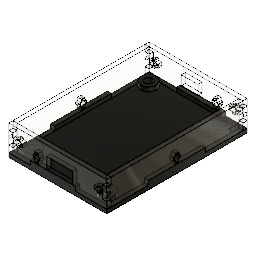
FinalProject_Enclosure_v2 (Autodesk Fusion 360 design; units mm, degrees)
Autodesk Fusion 360 part; units mm, degrees
(part 1 of 2)
sketch "Sketch1" plane through (0, 0, 0) normal (0, 0, 1) x (1, 0, 0) in component "Internals"
  line L0 (31.75, 47) -> (-31.75, 47)
  line L1 (-31.75, 47) -> (-31.75, -47)
  line L2 (-31.75, -47) -> (31.75, -47)
  line L3 (31.75, -47) -> (31.75, 47)
  line L4 (31.75, 47) -> (-31.75, -47) construction
  line L5 (-31.75, 47) -> (31.75, -47) construction
  line L6 (50.5, 1.5) -> (-50.5, 1.5) construction
  line L7 (-50.5, 1.5) -> (-50.5, -4.5) construction
  line L8 (-50.5, -4.5) -> (50.5, -4.5) construction
  line L9 (50.5, -4.5) -> (50.5, 1.5) construction
  line L10 (0, -50.5) -> (0, 50.5) construction
  point P0 (-33.75, 0)
  point P1 (33.75, 0)
  constraint horizontal L0
  constraint perpendicular L0 L1
  constraint parallel L0 L2
  constraint parallel L1 L3
  constraint coincident L4 origin
  constraint coincident L5 origin
  measures "d16" distance of L1.end L2.end
  measures "d17" distance of L0.end L1.end
extrude "Extrude1" add sketch "Sketch1" along normal blind 1.5 makes body 1 in component "Internals"
sketch "Sketch2" plane through (0, 0, 1.5) normal (0, 0, 1) x (-1, 0, 0) in component "Internals"
  line L0 (-31.75, 47) -> (-31.75, -47)
  line L1 (-31.75, -47) -> (31.75, -47)
  line L2 (31.75, -47) -> (31.75, 47)
  line L3 (31.75, 47) -> (-31.75, 47)
  line L4 (31.75, -41) -> (-31.75, -41) construction
  line L5 (25.75, -47) -> (25.75, 47) construction
  line L6 (0, -47) -> (0, 47) construction
  line L7 (31.75, 0) -> (-31.75, 0) construction
  line L8 (31.75, 41) -> (-31.75, 41) construction
  line L9 (-25.75, -47) -> (-25.75, 47) construction
  circle A0 centre (25.75, 41) radius 1.5
  circle A1 centre (-25.75, 41) radius 1.5
  circle A2 centre (-25.75, -41) radius 1.5
  circle A3 centre (25.75, -41) radius 1.5
  dimension "d20" = 6
  dimension "d21" = 6
  dimension "d22" = 3
  dimension "d23" = 3
  dimension "d24" = 3
  dimension "d25" = 3
  constraint coincident L2 L4.start
  constraint coincident L0 L4.end
  constraint perpendicular L0 L4
  constraint coincident L1 L5.start
  constraint coincident L3 L5.end
  constraint perpendicular L3 L5
  constraint midpoint L1 L6.start
  constraint midpoint L3 L6.end
  constraint midpoint L2 L7.start
  constraint midpoint L0 L7.end
  constraint symmetric L4.start L7 L8.start
  constraint symmetric L4.end L7 L8.end
  constraint symmetric L5.start L6 L9.start
  constraint symmetric L5.end L6 L9.end
  constraint coincident L5 A0.centre
  constraint coincident L8 A0.centre
  constraint coincident L9 A1.centre
  constraint coincident L8 A1.centre
  constraint coincident L9 A2.centre
  constraint coincident L4 A2.centre
  constraint coincident L5 A3.centre
  constraint coincident L4 A3.centre
  measures "d20" distance of L1 L4
  measures "d21" distance of L2 L5
  measures "d22" diameter of A0
  measures "d23" diameter of A1
  measures "d24" diameter of A2
  measures "d25" diameter of A3
extrude "Extrude2" add sketch "Sketch2" along normal blind 14 contours A0 | A1 | A2 | A3 bodies 1 in component "Internals"
sketch "Sketch3" plane through (0, 0, 15.5) normal (0, 0, 1) x (-1, 0, 0) in component "Internals"
  circle A0 centre (25.75, 41) radius 1.5
  line L0 (-31.75, -47) -> (31.75, -47)
  line L1 (31.75, -47) -> (31.75, 47)
  line L2 (31.75, 47) -> (-31.75, 47)
  line L3 (-31.75, 47) -> (-31.75, -47)
  line L4 (-31.75, -47) -> (31.75, 47) construction
  line L5 (31.75, -47) -> (-31.75, 47) construction
  dimension "d28" = 63.5
  dimension "d29" = 94
  constraint horizontal L0
  constraint perpendicular L0 L1
  constraint parallel L0 L2
  constraint parallel L1 L3
  constraint coincident L4 origin
  constraint coincident L5 origin
  measures "d28" distance of L1.end L2.end
  measures "d29" distance of L0.end L1.end
extrude "Extrude3" add sketch "Sketch3" along normal blind 1.5 contours A0 | L0 L1 L2 L3 bodies 1 in component "Internals"
sketch "Sketch4" plane through (0, 0, 17) normal (0, 0, 1) x (-1, 0, 0) in component "Internals"
  line L0 (-31.75, 47) -> (-31.75, -47)
  line L1 (-31.75, -47) -> (31.75, -47)
  line L2 (31.75, -47) -> (31.75, 47)
  line L3 (31.75, 47) -> (-31.75, 47)
  line L4 (0, 47) -> (0, -47) construction
  line L5 (-31.75, 0) -> (31.75, 0) construction
  line L6 (-31.75, 1) -> (31.75, 1) construction
  line L7 (-5, 47) -> (-5, -47) construction
  line L8 (-5, 1) -> (-17.1, 1)
  line L9 (-17.1, 1) -> (-17.1, 13.1)
  line L10 (-17.1, 13.1) -> (-5, 13.1)
  line L11 (-5, 13.1) -> (-5, 1)
  line L12 (-17.1, 27.2) -> (-5, 27.2)
  line L13 (-17.1, 15.1) -> (-17.1, 27.2)
  line L14 (-5, 15.1) -> (-17.1, 15.1)
  line L15 (-5, 27.2) -> (-5, 15.1)
  line L16 (-17.1, -13.1) -> (-17.1, -1)
  line L17 (-17.1, -1) -> (-5, -1)
  line L18 (-5, -1) -> (-5, -13.1)
  line L19 (-5, -13.1) -> (-17.1, -13.1)
  line L20 (-17.1, -15.1) -> (-5, -15.1)
  line L21 (-17.1, -27.2) -> (-17.1, -15.1)
  line L22 (-5, -27.2) -> (-17.1, -27.2)
  line L23 (-5, -15.1) -> (-5, -27.2)
  line L24 (17.1, 27.2) -> (5, 27.2)
  line L25 (17.1, 15.1) -> (17.1, 27.2)
  line L26 (5, 15.1) -> (17.1, 15.1)
  line L27 (5, 27.2) -> (5, 15.1)
  line L28 (5, 13.1) -> (5, 1)
  line L29 (5, -1) -> (5, -13.1)
  line L30 (5, -15.1) -> (5, -27.2)
  line L31 (5, -27.2) -> (17.1, -27.2)
  line L32 (17.1, -27.2) -> (17.1, -15.1)
  line L33 (17.1, -15.1) -> (5, -15.1)
  line L34 (5, -13.1) -> (17.1, -13.1)
  line L35 (17.1, -13.1) -> (17.1, -1)
  line L36 (17.1, -1) -> (5, -1)
  line L37 (17.1, 1) -> (17.1, 13.1)
  line L38 (17.1, 13.1) -> (5, 13.1)
  line L39 (5, 1) -> (17.1, 1)
  line L40 (13, -29.2) -> (9.1, -29.2)
  line L41 (9.1, -29.2) -> (9.1, -41.1)
  line L42 (9.1, -41.1) -> (13, -41.1)
  line L43 (13, -41.1) -> (13, -29.2)
  line L44 (11.05, -15.1) -> (11.05, -53.5543) construction
  line L45 (11.05, -29.2) -> (11.05, -41.1) construction
  dimension "d32" = 1
  dimension "d33" = 5
  dimension "d34" = 12.1
  dimension "d35" = 12.1
  dimension "d36" = 12.1
  dimension "d37" = 12.1
  dimension "d38" = 12.1
  dimension "d39" = 12.1
  dimension "d40" = 12.1
  dimension "d41" = 12.1
  dimension "d42" = 3.9
  dimension "d43" = 11.9
  dimension "d44" = 2
  constraint midpoint L3 L4.start
  constraint midpoint L1 L4.end
  constraint midpoint L0 L5.start
  constraint midpoint L2 L5.end
  constraint coincident L0 L6.start
  constraint coincident L2 L6.end
  constraint perpendicular L2 L6
  constraint coincident L3 L7.start
  constraint coincident L1 L7.end
  constraint perpendicular L1 L7
  constraint horizontal L8
  constraint vertical L9
  constraint horizontal L10
  constraint vertical L11
  constraint coincident L6 L8.start
  constraint coincident L7 L8.start
  constraint horizontal L14
  constraint vertical L13
  constraint horizontal L12
  constraint vertical L15
  constraint horizontal L19
  constraint vertical L16
  constraint horizontal L17
  constraint vertical L18
  constraint horizontal L22
  constraint vertical L21
  constraint horizontal L20
  constraint vertical L23
  constraint symmetric L4 L8.start L28.end
  constraint symmetric L4 L8.end L37.start
  constraint symmetric L4 L9.end L37.end
  constraint symmetric L4 L10.end L28.start
  constraint symmetric L4 L12.start L24.start
  constraint symmetric L4 L12.end L24.end
  constraint symmetric L4 L14.start L26.start
  constraint symmetric L4 L13.start L25.start
  constraint symmetric L4 L16.end L35.end
  constraint symmetric L4 L17.end L29.start
  constraint symmetric L4 L18.end L29.end
  constraint symmetric L4 L16.start L34.end
  constraint symmetric L4 L21.start L31.end
  constraint symmetric L4 L20.end L30.start
  constraint symmetric L4 L22.start L30.end
  constraint symmetric L4 L20.start L32.end
  constraint horizontal L40
  constraint vertical L41
  constraint horizontal L42
  constraint vertical L43
  constraint midpoint L33 L44.start
  constraint perpendicular L1 L44
  constraint midpoint L40 L45.start
  constraint midpoint L42 L45.end
  constraint collinear L44 L45
  measures "d32" distance of L5 L6
  measures "d33" distance of L4 L7
  measures "d34" distance of L8.start L8.end
  measures "d35" distance of L8.start L10.end
  measures "d36" distance of L14.start L13.start
  measures "d37" distance of L12.end L14.start
  measures "d38" distance of L18.end L16.start
  measures "d39" distance of L17.end L18.end
  measures "d40" distance of L21.start L22.start
  measures "d41" distance of L20.end L22.start
  measures "d42" distance of L40.start L40.end
  measures "d43" distance of L40.start L42.end
  measures "d44" distance of L31 L40
extrude "Extrude4" add sketch "Sketch4" along normal blind 5.2 contours L40 L41 L42 L43 bodies 1 in component "Internals"
extrude "Extrude5" add sketch "Sketch4" along normal blind 6.4 contours L8 L9 L10 L11 | L12 L13 L14 L15 | L16 L17 L18 L19 | L20 L21 L22 L23 | L24 L25 L26 L27 | L28 L37 L38 L39 | L29 L34 L35 L36 | L30 L31 L32 L33 bodies 1 in component "Internals"
sketch "Sketch1 (2)" plane through (-31.75, 0, 0) normal (-1, 0, 0) x (0, -1, 0) in component "Long Side"
  line L0 (-47, 15.5) -> (47, 15.5)
  line L1 (47, 15.5) -> (47, 17)
  line L2 (47, 17) -> (-47, 17)
  line L3 (-47, 17) -> (-47, 15.5)
  line L4 (50.5, 1.5) -> (-50.5, 1.5) construction
  line L5 (-50.5, 1.5) -> (-50.5, -4.5) construction
  line L6 (-50.5, -4.5) -> (50.5, -4.5) construction
  line L7 (50.5, -4.5) -> (50.5, 1.5) construction
  line L8 (50.5, 1.5) -> (50.5, 32.1442) construction
  line L9 (-50.5, 1.5) -> (-50.5, 33.8603) construction
  line L10 (-50.5, 1.5) -> (50.5, 1.5)
  line L11 (50.5, 1.5) -> (50.5, 17)
  line L12 (50.5, 17) -> (-50.5, 17)
  line L13 (-50.5, 17) -> (-50.5, 1.5)
  line L14 (-50.5, 1.5) -> (-20.41, 1.5)
  line L15 (-20.41, 1.5) -> (-20.41, -1.5)
  line L16 (-20.41, -1.5) -> (-50.5, -1.5)
  line L17 (-50.5, -1.5) -> (-50.5, 1.5)
  line L18 (0, 30) -> (0, -21) construction
  line L19 (50.5, 1.5) -> (20.41, 1.5)
  line L20 (20.41, 1.5) -> (20.41, -1.5)
  line L21 (20.41, -1.5) -> (50.5, -1.5)
  line L22 (50.5, -1.5) -> (50.5, 1.5)
  line L23 (-1.25, 1.5) -> (1.25, 1.5)
  line L24 (1.25, 1.5) -> (1.25, 8.5)
  line L25 (1.25, 8.5) -> (-1.25, 8.5)
  line L26 (-1.25, 8.5) -> (-1.25, 1.5)
  line L27 (-2.45, 6.3) -> (2.45, 6.3)
  line L28 (2.45, 6.3) -> (2.45, 4.4)
  line L29 (2.45, 4.4) -> (-2.45, 4.4)
  line L30 (-2.45, 4.4) -> (-2.45, 6.3)
  line L31 (50.5, 17) -> (47.5, 17)
  line L32 (47.5, 17) -> (47.5, 12.375)
  line L33 (47.5, 12.375) -> (50.5, 12.375)
  line L34 (50.5, 12.375) -> (50.5, 17)
  line L35 (50.5, -1.5) -> (47.5, -1.5)
  line L36 (47.5, -1.5) -> (47.5, 3.125)
  line L37 (47.5, 3.125) -> (50.5, 3.125)
  line L38 (50.5, 3.125) -> (50.5, -1.5)
  circle A0 centre (49, 7.75) radius 1.25
  line L39 (50.5, 12.375) -> (47.5, 3.125) construction
  line L40 (-50.5, -1.5) -> (-47.5, -1.5)
  line L41 (-47.5, -1.5) -> (-47.5, 3.125)
  line L42 (-47.5, 3.125) -> (-50.5, 3.125)
  line L43 (-50.5, 3.125) -> (-50.5, -1.5)
  line L44 (-50.5, 17) -> (-47.5, 17)
  line L45 (-47.5, 17) -> (-47.5, 12.375)
  line L46 (-47.5, 12.375) -> (-50.5, 12.375)
  line L47 (-50.5, 12.375) -> (-50.5, 17)
  line L48 (-47.5, 12.375) -> (-50.5, 3.125) construction
  circle A1 centre (-49, 7.75) radius 1.25
  point P0 (0, 1.5)
  point P1 (0, 4.4)
  dimension "d61" = 101
  dimension "d62" = 15.5
  dimension "d63" = 30.09
  dimension "d64" = 3
  dimension "d71" = 2.5
  dimension "d72" = 7
  dimension "d73" = 4.9
  dimension "d74" = 1.9
  dimension "d75" = 2.9
  dimension "d77" = 3
  dimension "d78" = 4.625
  dimension "d79" = 3
  dimension "d80" = 4.625
  dimension "d81" = 2.5
  dimension "d82" = 3
  dimension "d83" = 4.625
  dimension "d84" = 3
  dimension "d85" = 4.625
  dimension "d86" = 2.5
  constraint coincident L4.start L7.end
  constraint perpendicular L4 L8
  constraint coincident L4.end L5.start
  constraint perpendicular L4 L9
  constraint horizontal L10
  constraint vertical L11
  constraint horizontal L12
  constraint vertical L13
  constraint horizontal L14
  constraint vertical L15
  constraint horizontal L16
  constraint vertical L17
  constraint vertical L18
  constraint symmetric L4.end L18 L4.start
  constraint symmetric L14.end L18 L19.end
  constraint symmetric L15.end L18 L20.end
  constraint symmetric L16.end L18 L21.end
  constraint horizontal L23
  constraint vertical L24
  constraint horizontal L25
  constraint vertical L26
  constraint coincident L10 L23.start
  constraint midpoint L23 P0
  constraint midpoint L10 P0
  constraint horizontal L27
  constraint vertical L28
  constraint horizontal L29
  constraint vertical L30
  constraint midpoint L29 P1
  constraint coincident L18 P1
  constraint horizontal L31
  constraint vertical L32
  constraint horizontal L33
  constraint vertical L34
  constraint horizontal L35
  constraint vertical L36
  constraint horizontal L37
  constraint vertical L38
  constraint midpoint A0.centre L39
  constraint horizontal L40
  constraint vertical L41
  constraint horizontal L42
  constraint vertical L43
  constraint horizontal L44
  constraint vertical L45
  constraint horizontal L46
  constraint vertical L47
  constraint midpoint L48 A1.centre
  measures "d61" distance of L4.end L4.start
  measures "d62" distance of L4.end L12.end
  measures "d63" distance of L4.end L14.end
  measures "d64" distance of L4.end L16.end
  measures "d71" distance of L23.start L23.end
  measures "d72" distance of L23.start L25.end
  measures "d73" distance of L27.start L27.end
  measures "d74" distance of L27.start L29.end
  measures "d75" distance of L10 L29
  measures "d77" distance of L11.end L31.end
  measures "d78" distance of L11.end L33.end
  measures "d79" distance of L21.end L35.end
  measures "d80" distance of L21.end L37.end
  measures "d81" diameter of A0
  measures "d82" distance of L16.end L40.end
  measures "d83" distance of L16.end L42.end
  measures "d84" distance of L12.end L44.end
  measures "d85" distance of L12.end L46.end
  measures "d86" diameter of A1
extrude "Extrude1'" add sketch "Sketch1 (2)" along normal blind 3 from surface at 0.5 separate body contours L0 L1 L2 L3 L12 | L0 L1 L3 L10 L11 L12 L13 L14 L19 L24 L25 L26 L27 L28 L29 L30 L32 L33 L36 L37 L41 L42 L45 L46 | L10 L14 L15 L16 L41 | L10 L19 L20 L21 L36 makes body 2 in component "Long Side"
sketch "Sketch1 (3)" plane through (0, 0, 0) normal (0, 0, -1) x (1, 0, 0) in component "Base"
  line L0 (31.75, -47) -> (31.75, 47)
  line L1 (31.75, 47) -> (-31.75, 47)
  line L2 (-31.75, 47) -> (-31.75, -47)
  line L3 (-31.75, -47) -> (31.75, -47)
  line L4 (-32.25, -47.5) -> (32.25, -47.5)
  line L5 (32.25, -47.5) -> (32.25, 47.5)
  line L6 (32.25, 47.5) -> (-32.25, 47.5)
  line L7 (-32.25, 47.5) -> (-32.25, -47.5)
  line L8 (-32.25, -47.5) -> (32.25, 47.5) construction
  line L9 (32.25, -47.5) -> (-32.25, 47.5) construction
  line L10 (-35.25, -50.5) -> (35.25, -50.5)
  line L11 (35.25, -50.5) -> (35.25, 50.5)
  line L12 (35.25, 50.5) -> (-35.25, 50.5)
  line L13 (-35.25, 50.5) -> (-35.25, -50.5)
  line L14 (-35.25, -50.5) -> (35.25, 50.5) construction
  line L15 (35.25, -50.5) -> (-35.25, 50.5) construction
  dimension "d49_1" = 64.5
  dimension "d50_1" = 95
  dimension "d53_1" = 70.5
  dimension "d54_1" = 101
  constraint horizontal L4
  constraint perpendicular L4 L5
  constraint parallel L4 L6
  constraint parallel L5 L7
  constraint coincident L8 origin
  constraint coincident L9 origin
  constraint horizontal L10
  constraint perpendicular L10 L11
  constraint parallel L10 L12
  constraint parallel L11 L13
  constraint coincident L14 origin
  constraint coincident L15 origin
  measures "d49_1" distance of L5.end L6.end
  measures "d50_1" distance of L4.end L5.end
  measures "d53_1" distance of L11.end L12.end
  measures "d54_1" distance of L10.end L11.end
extrude "Extrude1''" add sketch "Sketch1 (3)" along normal blind 6 from surface at -1.5 separate body contours L10 L11 L12 L13 makes body 3 in component "Base"
extrude "Extrude2'" add sketch "Sketch1 (3)" along normal blind 3 from surface at 1.5 contours L0 L1 L2 L3 | L4 L5 L6 L7 bodies 3 in component "Base"
sketch "Sketch2 (2)" plane through (0, 0, 1.5) normal (0, 0, 1) x (-1, 0, 0) in component "Base"
  line L0 (32.25, 47.5) -> (32.25, -47.5)
  line L1 (32.25, -47.5) -> (-32.25, -47.5)
  line L2 (-32.25, -47.5) -> (-32.25, 47.5)
  line L3 (-32.25, 47.5) -> (32.25, 47.5)
  line L4 (35.25, -50.5) -> (35.25, 50.5)
  line L5 (35.25, 50.5) -> (-35.25, 50.5)
  line L6 (-35.25, 50.5) -> (-35.25, -50.5)
  line L7 (-35.25, -50.5) -> (35.25, -50.5)
  line L8 (32.25, -47.75) -> (32.25, -50.25)
  line L9 (32.25, 50.25) -> (32.25, 47.75)
  line L10 (32.25, -47.5) -> (32.25, 47.5)
  line L11 (32.25, 47.5) -> (32.25, 50.5)
  line L12 (32.25, 50.5) -> (32.25, 47.5)
  line L13 (32.25, 47.5) -> (32.25, 20.41)
  line L14 (32.25, 20.41) -> (32.25, 1.25)
  line L15 (32.25, 1.25) -> (32.25, 2.45)
  line L16 (32.25, 2.45) -> (32.25, 1.25)
  line L17 (32.25, 1.25) -> (32.25, -1.25)
  line L18 (32.25, -1.25) -> (32.25, -2.45)
  line L19 (32.25, -2.45) -> (32.25, -1.25)
  line L20 (32.25, -1.25) -> (32.25, -20.41)
  line L21 (32.25, -20.41) -> (32.25, -47.5)
  line L22 (32.25, -47.5) -> (32.25, -50.5)
  line L23 (32.25, -50.5) -> (32.25, -47.5)
  line L24 (35.25, -50.5) -> (32.25, -50.5)
  line L25 (32.25, -50.5) -> (32.25, -20.41)
  line L26 (32.25, -20.41) -> (35.25, -20.41)
  line L27 (35.25, -20.41) -> (35.25, -50.5)
  line L28 (35.25, 50.5) -> (32.25, 50.5)
  line L29 (32.25, 50.5) -> (32.25, 20.41)
  line L30 (32.25, 20.41) -> (35.25, 20.41)
  line L31 (35.25, 20.41) -> (35.25, 50.5)
  line L32 (35.25, -20.41) -> (32.25, 20.41) construction
  circle A0 centre (33.75, 0) radius 1.25
  line L33 (0, -50.5) -> (0, 50.5) construction
  line L34 (32.25, -20.41) -> (-35.25, -20.41) construction
  line L35 (32.25, 20.41) -> (-35.25, 20.41) construction
  line L36 (-35.25, -50.5) -> (-32.25, -50.5)
  line L37 (-32.25, -50.5) -> (-32.25, -20.41)
  line L38 (-32.25, -20.41) -> (-35.25, -20.41)
  line L39 (-35.25, -20.41) -> (-35.25, -50.5)
  line L40 (-35.25, 50.5) -> (-32.25, 50.5)
  line L41 (-32.25, 50.5) -> (-32.25, 20.41)
  line L42 (-32.25, 20.41) -> (-35.25, 20.41)
  line L43 (-35.25, 20.41) -> (-35.25, 50.5)
  line L44 (-35.25, -20.41) -> (-32.25, 20.41) construction
  circle A1 centre (-33.75, 0) radius 1.25
  line L45 (-35.25, -50.5) -> (-19.75, -50.5)
  line L46 (-19.75, -50.5) -> (-19.75, -47.5)
  line L47 (-19.75, -47.5) -> (-35.25, -47.5)
  line L48 (-35.25, -47.5) -> (-35.25, -50.5)
  line L49 (35.25, -50.5) -> (12.75, -50.5)
  line L50 (12.75, -50.5) -> (12.75, -47.5)
  line L51 (12.75, -47.5) -> (35.25, -47.5)
  line L52 (35.25, -47.5) -> (35.25, -50.5)
  line L53 (-35.25, 50.5) -> (-12.75, 50.5)
  line L54 (-12.75, 50.5) -> (-12.75, 47.5)
  line L55 (-12.75, 47.5) -> (-35.25, 47.5)
  line L56 (-35.25, 47.5) -> (-35.25, 50.5)
  line L57 (35.25, 50.5) -> (19.75, 50.5)
  line L58 (19.75, 50.5) -> (19.75, 47.5)
  line L59 (19.75, 47.5) -> (35.25, 47.5)
  line L60 (35.25, 47.5) -> (35.25, 50.5)
  circle A2 centre (-15.25, -49) radius 1.25
  circle A3 centre (15.25, 49) radius 1.25
  point P0 (35.25, -20.41)
  dimension "d90" = 2.5
  dimension "d91" = 2.5
  dimension "d121" = 15.5
  dimension "d122" = 3
  dimension "d123" = 22.5
  dimension "d124" = 3
  dimension "d125" = 22.5
  dimension "d126" = 3
  dimension "d127" = 15.5
  dimension "d128" = 3
  dimension "d129" = 2.5
  dimension "d130" = 2.5
  dimension "d150" = 4.5
  dimension "d151" = 4.5
  constraint horizontal L24
  constraint vertical L25
  constraint horizontal L26
  constraint vertical L27
  constraint coincident L20.end L21.start
  constraint coincident L4.start L7.end
  constraint horizontal L28
  constraint vertical L29
  constraint horizontal L30
  constraint vertical L31
  constraint coincident L13.end L14.start
  constraint coincident L4.end L5.start
  constraint coincident P0 L26.end
  constraint midpoint L32 A0.centre
  constraint midpoint L7 L33.start
  constraint midpoint L5 L33.end
  constraint coincident L6 L34.end
  constraint perpendicular L6 L34
  constraint coincident L6 L35.end
  constraint perpendicular L6 L35
  constraint horizontal L36
  constraint vertical L37
  constraint horizontal L38
  constraint vertical L39
  constraint coincident L2 L37.end
  constraint coincident L34 L37.end
  constraint coincident L6.end L7.start
  constraint horizontal L40
  constraint vertical L41
  constraint horizontal L42
  constraint vertical L43
  constraint coincident L35 L41.end
  constraint coincident L2 L41.end
  constraint coincident L5.end L6.start
  constraint midpoint L44 A1.centre
  constraint horizontal L45
  constraint vertical L46
  constraint horizontal L47
  constraint vertical L48
  constraint horizontal L49
  constraint vertical L50
  constraint horizontal L51
  constraint vertical L52
  constraint horizontal L53
  constraint vertical L54
  constraint horizontal L55
  constraint vertical L56
  constraint horizontal L57
  constraint vertical L58
  constraint horizontal L59
  constraint vertical L60
  measures "d90" diameter of A0
  measures "d91" diameter of A1
  measures "d121" distance of L6.end L45.end
  measures "d122" distance of L6.end L47.end
  measures "d123" distance of L4.start L49.end
  measures "d124" distance of L4.start L51.end
  measures "d125" distance of L5.end L53.end
  measures "d126" distance of L5.end L55.end
  measures "d127" distance of L4.end L57.end
  measures "d128" distance of L4.end L59.end
  measures "d129" diameter of A2
  measures "d130" diameter of A3
  measures "d150" distance of L46 A2.centre
  measures "d151" distance of L58 A3.centre
extrude "Extrude3'" cut sketch "Sketch2 (2)" against normal blind 3 contours L0 L4 L10 L13 L29 L30 L31 L59 | L3 L5 L9 L11 L12 L29 L57 L58 L59 | L4 L5 L9 L11 L12 L28 L29 L31 L57 L59 L60 | L3 L5 L41 L53 L54 L55 | L0 L4 L10 L21 L25 L26 L27 L51 | L5 L6 L40 L41 L43 L53 L55 L56 | L2 L6 L41 L42 L43 L55 | L4 L7 L8 L22 L23 L24 L25 L27 L49 L51 L52 | L1 L7 L8 L22 L23 L25 L49 L50 L51 | L2 L6 L37 L38 L39 L47 | L1 L7 L37 L45 L46 L47 | L6 L7 L36 L37 L39 L45 L47 L48 bodies 3 in component "Base"
extrude "Extrude4'" cut sketch "Sketch2 (2)" against normal blind 14 contours A0 | A1 | A2 | A3 bodies 3 in component "Base"
sketch "Sketch1 (4)" plane through (0, 47, 0) normal (0, 1, 0) x (-1, 0, 0) in component "Short Side"
  line L0 (-31.75, 15.5) -> (31.75, 15.5)
  line L1 (31.75, 15.5) -> (31.75, 17)
  line L2 (31.75, 17) -> (-31.75, 17)
  line L3 (-31.75, 17) -> (-31.75, 15.5)
  line L4 (12.75, 1.5) -> (-19.75, 1.5)
  line L5 (-19.75, -1.5) -> (-35.25, -1.5)
  line L6 (-35.25, -1.5) -> (-35.25, -4.5)
  line L7 (-35.25, -4.5) -> (35.25, -4.5)
  line L8 (35.25, -4.5) -> (35.25, -1.5)
  line L9 (35.25, -1.5) -> (12.75, -1.5)
  line L10 (35.25, -4.5) -> (35.25, 23) construction
  line L11 (-35.25, -1.5) -> (35.25, -1.5)
  line L12 (35.25, -1.5) -> (35.25, 17)
  line L13 (35.25, 17) -> (-35.25, 17)
  line L14 (-35.25, 17) -> (-35.25, -1.5)
  line L15 (35.25, 17) -> (32.25, 17)
  line L16 (32.25, 12.195) -> (35.25, 12.195)
  line L17 (35.25, 12.195) -> (35.25, 17)
  line L18 (35.25, -1.5) -> (32.25, -1.5)
  line L19 (32.25, 3.305) -> (35.25, 3.305)
  line L20 (35.25, 3.305) -> (35.25, -1.5)
  line L21 (-35.25, 17) -> (-32.25, 17)
  line L22 (-32.25, 12.195) -> (-35.25, 12.195)
  line L23 (-35.25, 12.195) -> (-35.25, 17)
  line L24 (-35.25, -1.5) -> (-32.25, -1.5)
  line L25 (-32.2728, 3.305) -> (-35.25, 3.305)
  line L26 (-35.25, 3.305) -> (-35.25, -1.5)
  line L27 (-32.2728, 3.305) -> (-35.25, 3.305)
  line L28 (-35.25, 3.305) -> (-35.25, 12.195)
  line L29 (-35.25, 12.195) -> (-32.2728, 12.195)
  line L30 (-32.2728, 12.195) -> (-32.2728, 3.305)
  line L31 (32.25, 3.305) -> (35.25, 3.305)
  line L32 (35.25, 3.305) -> (35.25, 12.195)
  line L33 (35.25, 12.195) -> (32.25, 12.195)
  line L34 (32.25, 12.195) -> (32.25, 3.305)
  line L35 (0.4382, 30) -> (0.4382, -14) construction
  line L36 (-9.5349, -1.5) -> (15.25, -1.5)
  line L37 (-0.8118, -1) -> (1.6882, -1)
  line L38 (35.25, 7.75) -> (-35.25, 7.75) construction
  line L39 (-32.2728, 9) -> (-25.2728, 9)
  line L40 (-25.2728, 9) -> (-25.2728, 6.5)
  line L41 (-25.2728, 6.5) -> (-32.2728, 6.5)
  line L42 (-32.2728, 6.5) -> (-32.2728, 9)
  line L43 (-27.4728, 10.2) -> (-29.3728, 10.2)
  line L44 (-29.3728, 10.2) -> (-29.3728, 5.3)
  line L45 (-29.3728, 5.3) -> (-27.4728, 5.3)
  line L46 (-27.4728, 5.3) -> (-27.4728, 10.2)
  line L47 (-27.4728, 10.2) -> (-29.3728, 5.3) construction
  line L48 (-29.3728, 10.2) -> (-27.4728, 5.3) construction
  line L49 (33.1492, 9) -> (26.1492, 9)
  line L50 (26.1492, 6.5) -> (33.1492, 6.5)
  line L51 (26.1492, 9) -> (26.1492, 6.5)
  line L52 (28.3492, 5.3) -> (28.3492, 10.2)
  line L53 (30.2492, 10.2) -> (30.2492, 5.3)
  line L54 (28.3492, 10.2) -> (30.2492, 10.2)
  line L55 (30.2492, 5.3) -> (28.3492, 5.3)
  line L56 (12.75, -1.5) -> (12.75, 1.5)
  line L57 (-19.75, 1.5) -> (-19.75, -1.5)
  line L58 (-15.25, 17) -> (-15.25, -1.5) construction
  line L59 (-19.66, 17) -> (-19.66, -1.5) construction
  line L60 (12.66, 17) -> (12.66, -1.5) construction
  line L61 (-14, 8.5) -> (-16.5, 8.5)
  line L62 (-16.5, 8.5) -> (-16.5, 1.5)
  line L63 (-16.5, 1.5) -> (-14, 1.5)
  line L64 (-14, 1.5) -> (-14, 8.5)
  line L65 (-14, 8.5) -> (-16.5, 1.5) construction
  line L66 (-16.5, 8.5) -> (-14, 1.5) construction
  line L67 (-12.8, 6.3) -> (-17.7, 6.3)
  line L68 (-17.7, 6.3) -> (-17.7, 4.4)
  line L69 (-17.7, 4.4) -> (-12.8, 4.4)
  line L70 (-12.8, 4.4) -> (-12.8, 6.3)
  line L71 (-12.8, 6.3) -> (-17.7, 4.4) construction
  line L72 (-17.7, 6.3) -> (-12.8, 4.4) construction
  line L73 (-2.75, 11) -> (9.25, 11)
  line L74 (9.25, 11) -> (9.25, 4)
  line L75 (9.25, 4) -> (-2.75, 4)
  line L76 (-2.75, 4) -> (-2.75, 11)
  line L77 (12.66, 1.5) -> (-19.66, 1.5)
  line L78 (-19.66, 1.5) -> (-19.66, -1.5)
  line L79 (-19.66, -1.5) -> (12.66, -1.5)
  line L80 (12.66, -1.5) -> (12.66, 1.5)
  point P0 (0.4382, -1)
  point P1 (0.4382, 5.5)
  point P2 (-32.2728, 7.75)
  point P3 (-28.4228, 7.75)
  point P4 (-15.25, 5)
  point P5 (-15.25, 1.5)
  point P6 (-15.25, 5.35)
  dimension "d96" = 70.5
  dimension "d97" = 18.5
  dimension "d98" = 3
  dimension "d99" = 4.805
  dimension "d100" = 3
  dimension "d101" = 4.805
  dimension "d102" = 3
  dimension "d103" = 4.805
  dimension "d104" = 3
  dimension "d105" = 4.805
  dimension "d108" = 2.5
  dimension "d113" = 7
  dimension "d114" = 2.5
  dimension "d115" = 1.9
  dimension "d116" = 4.9
  dimension "d117" = 2.9
  dimension "d152" = 20
  dimension "d153" = 15.59
  dimension "d154" = 22.59
  dimension "d155" = 7
  dimension "d156" = 4.9
  dimension "d157" = 1.9
  dimension "d159" = 12
  dimension "d160" = 7
  dimension "d162" = 26
  dimension "d163" = 32.5
  dimension "d180" = 6
  dimension "d184" = 2.9
  dimension "d185" = 2.5
  constraint coincident L7.end L8.start
  constraint perpendicular L7 L10
  constraint horizontal L11
  constraint vertical L12
  constraint horizontal L13
  constraint vertical L14
  constraint coincident L5.end L6.start
  constraint horizontal L15
  constraint horizontal L16
  constraint vertical L17
  constraint horizontal L18
  constraint horizontal L19
  constraint vertical L20
  constraint coincident L8.end L9.start
  constraint horizontal L21
  constraint horizontal L22
  constraint vertical L23
  constraint horizontal L24
  constraint horizontal L25
  constraint vertical L26
  constraint horizontal L27
  constraint vertical L28
  constraint horizontal L29
  constraint vertical L30
  constraint horizontal L31
  constraint vertical L32
  constraint horizontal L33
  constraint vertical L34
  constraint vertical L35
  constraint horizontal L36
  constraint coincident L11 L36.start
  constraint horizontal L37
  constraint midpoint L37 P0
  constraint vertical L35.end P0
  constraint coincident L35 P1
  constraint midpoint L12 L38.start
  constraint midpoint L28 L38.end
  constraint horizontal L39
  constraint vertical L40
  constraint horizontal L41
  constraint vertical L42
  constraint coincident L30 L39.start
  constraint midpoint L42 P2
  constraint horizontal L38.end P2
  constraint horizontal L43
  constraint perpendicular L43 L44
  constraint parallel L43 L45
  constraint parallel L44 L46
  constraint coincident L47 P3
  constraint coincident L48 P3
  constraint coincident L38 P3
  constraint symmetric L35 L39.start L49.start
  constraint symmetric L35 L39.end L49.end
  constraint symmetric L35 L40.end L50.start
  constraint symmetric L35 L41.end L50.end
  constraint symmetric L35 L43.start L52.end
  constraint symmetric L35 L43.end L53.start
  constraint symmetric L35 L44.end L53.end
  constraint symmetric L35 L45.end L52.start
  constraint coincident L13 L58.start
  constraint coincident L11 L58.end
  constraint perpendicular L11 L58
  constraint coincident L2 L59.start
  constraint coincident L11 L59.end
  constraint perpendicular L11 L59
  constraint coincident L13 L60.start
  constraint coincident L36 L60.end
  constraint perpendicular L36 L60
  constraint horizontal L61
  constraint perpendicular L61 L62
  constraint parallel L61 L63
  constraint parallel L62 L64
  constraint coincident L65 P4
  constraint coincident L66 P4
  constraint coincident L58 P4
  constraint coincident L63 P5
  constraint horizontal L67
  constraint perpendicular L67 L68
  constraint parallel L67 L69
  constraint parallel L68 L70
  constraint coincident L71 P6
  constraint coincident L72 P6
  constraint coincident L58 P6
  constraint horizontal L73
  constraint vertical L74
  constraint horizontal L75
  constraint vertical L76
  constraint horizontal L77
  constraint vertical L78
  constraint horizontal L79
  constraint vertical L80
  constraint coincident L60 L77.start
  constraint coincident L4 L77.start
  measures "d96" distance of L5.end L8.end
  measures "d97" distance of L5.end L13.end
  measures "d98" distance of L12.end L15.end
  measures "d99" distance of L12.end L16.end
  measures "d100" distance of L8.end L18.end
  measures "d101" distance of L8.end L19.end
  measures "d102" distance of L13.end L21.end
  measures "d103" distance of L13.end L22.end
  measures "d104" distance of L5.end L24.end
  measures "d105" distance of L5.end L25.end
  measures "d108" distance of L37.start L37.end
  measures "d113" distance of L39.start L39.end
  measures "d114" distance of L39.start L41.end
  measures "d115" distance of L44.end L45.end
  measures "d116" distance of L43.end L44.end
  measures "d117" distance of L30 L44
  measures "d152" distance of L14 L58
  measures "d153" distance of L23 L59
  measures "d154" distance of L10 L60
  measures "d155" distance of L61.end L62.end
  measures "d156" distance of L68.end L69.end
  measures "d157" distance of L67.end L68.end
  measures "d159" distance of L73.start L73.end
  measures "d160" distance of L73.start L75.end
  measures "d162" distance of L12 L74
  measures "d163" distance of L23 L76
  measures "d180" distance of L13 L73
  measures "d184" distance of L69.end L77
  measures "d185" distance of L61.start L61.end
sketch "Sketch3 (2)" plane through (0, 0, -1.5) normal (0, 0, 1) x (-1, 0, 0) in component "Base"
  line L0 (19.75, 47.5) -> (-12.75, 47.5)
  line L1 (-12.75, 47.5) -> (-12.75, 50.5)
  line L2 (-12.75, 50.5) -> (-35.25, 50.5)
  line L3 (-35.25, 50.5) -> (-35.25, 20.41)
  line L4 (-35.25, 20.41) -> (-32.25, 20.41)
  line L5 (-32.25, 20.41) -> (-32.25, -20.41)
  line L6 (-32.25, -20.41) -> (-35.25, -20.41)
  line L7 (-35.25, -20.41) -> (-35.25, -50.5)
  line L8 (-35.25, -50.5) -> (-19.75, -50.5)
  line L9 (-19.75, -50.5) -> (-19.75, -47.5)
  line L10 (-19.75, -47.5) -> (12.75, -47.5)
  line L11 (12.75, -47.5) -> (12.75, -50.5)
  line L12 (12.75, -50.5) -> (35.25, -50.5)
  line L13 (35.25, -50.5) -> (35.25, -20.41)
  line L14 (35.25, -20.41) -> (32.25, -20.41)
  line L15 (32.25, -20.41) -> (32.25, 20.41)
  line L16 (32.25, 20.41) -> (35.25, 20.41)
  line L17 (35.25, 20.41) -> (35.25, 50.5)
  line L18 (35.25, 50.5) -> (19.75, 50.5)
  line L19 (19.75, 50.5) -> (19.75, 47.5)
  circle A0 centre (-26.75, 41.5) radius 5.5
  line L20 (-12.75, 47.5) -> (-35.25, 47.5)
  line L21 (-32.25, 50.5) -> (-32.25, 20.41)
  line L22 (15.25, 49) -> (-15.25, -49) construction
  line L23 (-33.75, 0) -> (33.75, 0) construction
  line L24 (0, -50.5) -> (0, 50.5) construction
  circle A1 centre (26.75, 41.5) radius 5.5
  circle A2 centre (26.75, -41.5) radius 5.5
  circle A3 centre (-26.75, -41.5) radius 5.5
  circle A4 centre (-26.75, 41.5) radius 2.75
  circle A5 centre (26.75, 41.5) radius 2.75
  circle A6 centre (26.75, -41.5) radius 2.75
  circle A7 centre (-26.75, -41.5) radius 2.75
  line L25 (19.75, 47.5) -> (35.25, 47.5)
  line L26 (32.25, 20.41) -> (32.25, 50.5)
  line L27 (32.25, -20.41) -> (32.25, -50.5)
  line L28 (12.75, -47.5) -> (35.25, -47.5)
  line L29 (-19.75, -47.5) -> (-35.25, -47.5)
  line L30 (-32.25, -20.41) -> (-32.25, -50.5)
  line L31 (-32.25, 41.5) -> (-32.25, 50.5)
  line L32 (-26.75, 41.5) -> (-26.75, 47) construction
  line L33 (-26.75, 47) -> (-35.25, 47)
  line L34 (26.75, 47) -> (35.25, 47)
  line L35 (32.25, 41.5) -> (32.25, 50.5)
  line L36 (-26.75, -47) -> (-35.25, -47)
  line L37 (-32.25, -41.5) -> (-32.25, -50.5)
  line L38 (26.75, -47) -> (35.25, -47)
  line L39 (32.25, -41.5) -> (32.25, -50.5)
  point P0 (15.25, 49)
  point P1 (-33.75, 0)
  point P2 (-15.25, -49)
  point P3 (33.75, 0)
  dimension "d133" = 11
  dimension "d134" = 6
  dimension "d135" = 5.5
  dimension "d136" = 5.5
  constraint coincident P0 L22.start
  constraint coincident P2 L22.end
  constraint coincident P1 L23.start
  constraint coincident P3 L23.end
  constraint symmetric A0 L24 A1
  constraint symmetric A0 L23 A3
  constraint symmetric L23 A1 A2
  constraint concentric A0 A4
  constraint symmetric L24 A4 A5
  constraint symmetric L23 A4 A7
  constraint symmetric L23 A5 A6
  constraint coincident L0.start L19.end
  constraint coincident L17 L25.end
  constraint perpendicular L17 L25
  constraint coincident L15.end L16.start
  constraint coincident L18 L26.end
  constraint perpendicular L18 L26
  constraint coincident L14.end L15.start
  constraint coincident L12 L27.end
  constraint perpendicular L12 L27
  constraint coincident L10.end L11.start
  constraint coincident L13 L28.end
  constraint perpendicular L13 L28
  constraint coincident L9.end L10.start
  constraint coincident L7 L29.end
  constraint perpendicular L7 L29
  constraint coincident L5.end L6.start
  constraint coincident L8 L30.end
  constraint perpendicular L8 L30
  constraint coincident A0 L31.start
  constraint coincident L21.start L31.end
  constraint tangent A0 L31
  constraint coincident A0.centre A4.centre
  constraint coincident A0 L32.end
  constraint vertical L32
  constraint coincident L3 L33.end
  constraint perpendicular L3 L33
  constraint symmetric L24 L31.start L35.start
  constraint symmetric L24 L21.start L26.end
  constraint symmetric L24 L32.end L34.start
  constraint symmetric L24 L33.end L34.end
  constraint symmetric L23 L31.start L37.start
  constraint symmetric L23 L21.start L30.end
  constraint symmetric L23 L32.end L36.start
  constraint symmetric L23 L33.end L36.end
  constraint symmetric L23 L34.start L38.start
  constraint symmetric L23 L34.end L38.end
  constraint symmetric L23 L35.start L39.start
  constraint symmetric L23 L26.end L27.end
  measures "d133" diameter of A0
  measures "d134" distance of A0.centre L20
  measures "d135" distance of A0.centre L21
  measures "d136" diameter of A4
sketch "Sketch1 (5)" plane through (0, 47, 0) normal (0, 1, 0) x (-1, 0, 0) in component "Short Side v1"
  line L0 (-31.75, 15.5) -> (31.75, 15.5)
  line L1 (31.75, 15.5) -> (31.75, 17)
  line L2 (31.75, 17) -> (-31.75, 17)
  line L3 (-31.75, 17) -> (-31.75, 15.5)
  line L4 (-35.25, -1.5454) -> (-35.25, -4.5)
  line L5 (-35.25, -4.5) -> (35.25, -4.5)
  line L6 (35.25, -4.5) -> (35.25, -1.5)
  line L7 (35.25, -4.5) -> (35.25, 23) construction
  line L8 (-35.25, -1.5454) -> (35.25, -1.5454)
  line L9 (35.25, -1.5454) -> (35.25, 16.9546)
  line L10 (35.25, 16.9546) -> (-35.25, 16.9546)
  line L11 (-35.25, 16.9546) -> (-35.25, -1.5454)
  line L12 (35.25, 16.9546) -> (32.25, 16.9546)
  line L13 (32.25, 12.1496) -> (35.25, 12.1496)
  line L14 (35.25, 12.1496) -> (35.25, 16.9546)
  line L15 (35.25, -1.5) -> (32.25, -1.5)
  line L16 (32.25, 3.305) -> (35.25, 3.305)
  line L17 (35.25, 3.305) -> (35.25, -1.5)
  line L18 (-35.25, 16.9546) -> (-32.25, 16.9546)
  line L19 (-32.25, 12.1496) -> (-35.25, 12.1496)
  line L20 (-35.25, 12.1496) -> (-35.25, 16.9546)
  line L21 (-35.25, -1.5454) -> (-32.25, -1.5454)
  line L22 (-32.3728, 3.2596) -> (-35.25, 3.2596)
  line L23 (-35.25, 3.2596) -> (-35.25, -1.5454)
  line L24 (-32.3728, 3.2596) -> (-35.25, 3.2596)
  line L25 (-35.25, 3.2596) -> (-35.25, 12.1496)
  line L26 (-35.25, 12.1496) -> (-32.3728, 12.1496)
  line L27 (-32.3728, 12.1496) -> (-32.3728, 3.2596)
  line L28 (32.25, 3.305) -> (35.25, 3.305)
  line L29 (35.25, 3.305) -> (35.25, 12.1496)
  line L30 (35.25, 12.1496) -> (32.25, 12.1496)
  line L31 (32.25, 12.1496) -> (32.25, 3.305)
  line L32 (0.4382, 30) -> (0.4382, -14) construction
  line L33 (-15.25, -1.5454) -> (15.25, -1.5454)
  line L34 (-0.8118, 1.45) -> (1.6882, 1.45)
  line L35 (35.25, 7.7046) -> (-35.25, 7.7046) construction
  line L36 (-32.3728, 8.9546) -> (-25.3728, 8.9546)
  line L37 (-25.3728, 8.9546) -> (-25.3728, 6.4546)
  line L38 (-25.3728, 6.4546) -> (-32.3728, 6.4546)
  line L39 (-32.3728, 6.4546) -> (-32.3728, 8.9546)
  line L40 (-27.5728, 10.1546) -> (-29.4728, 10.1546)
  line L41 (-29.4728, 10.1546) -> (-29.4728, 5.2546)
  line L42 (-29.4728, 5.2546) -> (-27.5728, 5.2546)
  line L43 (-27.5728, 5.2546) -> (-27.5728, 10.1546)
  line L44 (-27.5728, 10.1546) -> (-29.4728, 5.2546) construction
  line L45 (-29.4728, 10.1546) -> (-27.5728, 5.2546) construction
  line L46 (33.2492, 8.9546) -> (26.2492, 8.9546)
  line L47 (26.2492, 6.4546) -> (33.2492, 6.4546)
  line L48 (26.2492, 8.9546) -> (26.2492, 6.4546)
  line L49 (28.4492, 5.2546) -> (28.4492, 10.1546)
  line L50 (30.3492, 10.1546) -> (30.3492, 5.2546)
  line L51 (28.4492, 10.1546) -> (30.3492, 10.1546)
  line L52 (30.3492, 5.2546) -> (28.4492, 5.2546)
  line L53 (-15.25, 16.9546) -> (-15.25, -1.5454) construction
  line L54 (-19.66, 17) -> (-19.66, -1.5454) construction
  line L55 (12.66, 16.9546) -> (12.66, -1.5454) construction
  line L56 (-14, 8.4546) -> (-16.5, 8.4546)
  line L57 (-16.5, 8.4546) -> (-16.5, 1.4546)
  line L58 (-16.5, 1.4546) -> (-14, 1.4546)
  line L59 (-14, 1.4546) -> (-14, 8.4546)
  line L60 (-14, 8.4546) -> (-16.5, 1.4546) construction
  line L61 (-16.5, 8.4546) -> (-14, 1.4546) construction
  line L62 (-12.8, 6.2546) -> (-17.7, 6.2546)
  line L63 (-17.7, 6.2546) -> (-17.7, 4.3546)
  line L64 (-17.7, 4.3546) -> (-12.8, 4.3546)
  line L65 (-12.8, 4.3546) -> (-12.8, 6.2546)
  line L66 (-12.8, 6.2546) -> (-17.7, 4.3546) construction
  line L67 (-17.7, 6.2546) -> (-12.8, 4.3546) construction
  line L68 (-7.85, 9.9546) -> (10.85, 9.9546)
  line L69 (10.85, 9.9546) -> (10.85, 1.4546)
  line L70 (10.85, 1.4546) -> (-7.85, 1.4546)
  line L71 (-7.85, 1.4546) -> (-7.85, 9.9546)
  line L72 (-19.66, -1.5454) -> (12.66, -1.5454)
  line L73 (12.66, -1.5454) -> (12.66, 1.4546)
  line L74 (12.66, 1.4546) -> (-19.66, 1.4546)
  line L75 (-19.66, 1.4546) -> (-19.66, -1.5454)
  point P0 (0.4382, 1.45)
  point P1 (0.4382, 5.5)
  point P2 (-32.3728, 7.7046)
  point P3 (-28.5228, 7.7046)
  point P4 (-15.25, 4.9546)
  point P5 (-15.25, 1.4546)
  point P6 (-15.25, 5.3046)
  dimension "d96_1" = 70.5
  dimension "d97_1" = 18.5
  dimension "d98_1" = 3
  dimension "d99_1" = 4.805
  dimension "d100_1" = 3
  dimension "d101_1" = 4.805
  dimension "d102_1" = 3
  dimension "d103_1" = 4.805
  dimension "d104_1" = 3
  dimension "d105_1" = 4.805
  dimension "d108_1" = 2.5
  dimension "d113_1" = 7
  dimension "d114_1" = 2.5
  dimension "d115_1" = 1.9
  dimension "d116_1" = 4.9
  dimension "d117_1" = 2.9
  dimension "d152_1" = 20
  dimension "d153_1" = 15.59
  dimension "d154_1" = 22.59
  dimension "d155_1" = 7
  dimension "d156_1" = 4.9
  dimension "d157_1" = 1.9
  dimension "d172" = 18.7
  dimension "d173" = 8.5
  dimension "d174" = 24.4
  dimension "d186" = 2.5
  dimension "d187" = 32.32
  dimension "d188" = 3
  dimension "d189" = 2.9
  constraint coincident L5.end L6.start
  constraint perpendicular L5 L7
  constraint horizontal L8
  constraint vertical L9
  constraint horizontal L10
  constraint vertical L11
  constraint coincident L4.start L8.start
  constraint horizontal L12
  constraint horizontal L13
  constraint vertical L14
  constraint horizontal L15
  constraint horizontal L16
  constraint vertical L17
  constraint coincident L6.end L15.start
  constraint horizontal L18
  constraint horizontal L19
  constraint vertical L20
  constraint horizontal L21
  constraint horizontal L22
  constraint vertical L23
  constraint horizontal L24
  constraint vertical L25
  constraint horizontal L26
  constraint vertical L27
  constraint horizontal L28
  constraint vertical L29
  constraint horizontal L30
  constraint vertical L31
  constraint vertical L32
  constraint horizontal L33
  constraint coincident L8 L33.start
  constraint horizontal L34
  constraint vertical L32.end P0
  constraint coincident L32 P1
  constraint midpoint L9 L35.start
  constraint midpoint L25 L35.end
  constraint horizontal L36
  constraint vertical L37
  constraint horizontal L38
  constraint vertical L39
  constraint coincident L27 L36.start
  constraint midpoint L39 P2
  constraint horizontal L35.end P2
  constraint horizontal L40
  constraint perpendicular L40 L41
  constraint parallel L40 L42
  constraint parallel L41 L43
  constraint coincident L44 P3
  constraint coincident L45 P3
  constraint coincident L35 P3
  constraint symmetric L32 L36.start L46.start
  constraint symmetric L32 L36.end L46.end
  constraint symmetric L32 L37.end L47.start
  constraint symmetric L32 L38.end L47.end
  constraint symmetric L32 L40.start L49.end
  constraint symmetric L32 L40.end L50.start
  constraint symmetric L32 L41.end L50.end
  constraint symmetric L32 L42.end L49.start
  constraint coincident L10 L53.start
  constraint perpendicular L8 L53
  constraint coincident L2 L54.start
  constraint coincident L8 L54.end
  constraint perpendicular L8 L54
  constraint coincident L10 L55.start
  constraint coincident L33 L55.end
  constraint perpendicular L33 L55
  constraint horizontal L56
  constraint perpendicular L56 L57
  constraint parallel L56 L58
  constraint parallel L57 L59
  constraint coincident L60 P4
  constraint coincident L61 P4
  constraint coincident L53 P4
  constraint coincident L58 P5
  constraint horizontal L62
  constraint perpendicular L62 L63
  constraint parallel L62 L64
  constraint parallel L63 L65
  constraint coincident L66 P6
  constraint coincident L67 P6
  constraint coincident L53 P6
  constraint horizontal L68
  constraint vertical L69
  constraint horizontal L70
  constraint vertical L71
  constraint horizontal L72
  constraint vertical L73
  constraint horizontal L74
  constraint vertical L75
  constraint coincident L55 L73.end
  constraint coincident L70 L73.end
  constraint coincident L58.end L74
  measures "d96_1" distance of L4.start L8.end
  measures "d97_1" distance of L4.start L10.end
  measures "d98_1" distance of L9.end L12.end
  measures "d99_1" distance of L9.end L13.end
  measures "d100_1" distance of L6.end L15.end
  measures "d101_1" distance of L6.end L16.end
  measures "d102_1" distance of L10.end L18.end
  measures "d103_1" distance of L10.end L19.end
  measures "d104_1" distance of L4.start L21.end
  measures "d105_1" distance of L4.start L22.end
  measures "d108_1" distance of L34.start L34.end
  measures "d113_1" distance of L36.start L36.end
  measures "d114_1" distance of L36.start L38.end
  measures "d115_1" distance of L41.end L42.end
  measures "d116_1" distance of L40.end L41.end
  measures "d117_1" distance of L27 L41
  measures "d152_1" distance of L11 L53
  measures "d153_1" distance of L20 L54
  measures "d154_1" distance of L7 L55
  measures "d155_1" distance of L56.end L57.end
  measures "d156_1" distance of L63.end L64.end
  measures "d157_1" distance of L62.end L63.end
  measures "d172" distance of L68.start L68.end
  measures "d173" distance of L68.start L70.end
  measures "d174" distance of L14 L69
  measures "d186" distance of L56.start L56.end
  measures "d187" distance of L54.end L55.end
  measures "d188" distance of L54.end L74.end
  measures "d189" distance of L64 L74
extrude "Extrude5'" add sketch "Sketch1 (4)" along normal blind 3 from surface at 0.5 separate body contours L0 L1 L2 L3 L13 | L0 L1 L3 L4 L5 L9 L11 L12 L13 L14 L15 L16 L17 L18 L19 L20 L21 L22 L23 L24 L25 L26 L27 L29 L30 L31 L33 L34 L36 L39 L40 L41 L43 L44 L45 L46 L49 L50 L51 L52 L53 L54 L55 L56 L57 L61 L62 L64 L67 L68 L69 L70 L77 makes body 4 in component "Short Side"
extrude "Extrude3''" add sketch "Sketch1 (5)" along normal blind 3 from surface at 0.5 separate body contours L0 L1 L3 L10 | L0 L1 L3 L6 L8 L9 L10 L11 L12 L13 L14 L16 L17 L18 L19 L20 L21 L22 L23 L24 L26 L27 L28 L30 L31 L33 L36 L37 L38 L40 L41 L42 L43 L46 L47 L48 L49 L50 L51 L52 L56 L57 L59 L62 L63 L64 L65 L68 L69 L71 L73 L74 L75 makes body 5 in component "Short Side v1"